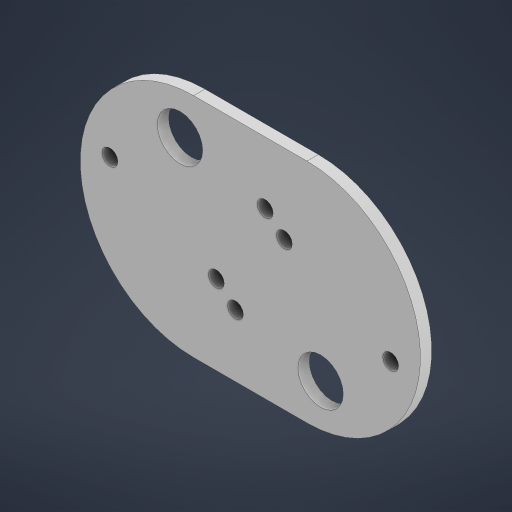
# Autodesk Inventor part: mount-plate
Saved by Autodesk Inventor 2024 (Build 280153000, 153)
## iProperties
Created: 2024-10-23
Part Number: mount-plate
Material: Generic
Document SubType Name: Modeling
Designer: loren
Density: 1 g/cm^3
Appearance: Default
Author: loren
## iProperties of the stored document mount-plate_3DPrint.ipt
Created: 2026-02-06
Part Number: mount-plate_3DPrint
Material: Generic
Document SubType Name: Modeling
Designer: lokies
Density: 1 g/cm^3
Appearance: Default
Author: lokies
Autodesk Inventor part; units mm, degrees
ref_plane "YZ Plane" through (0, 0, 0) normal (1, 0, 0) x (0, 1, 0)
ref_plane "XZ Plane" through (0, 0, 0) normal (0, 1, 0) x (-1, 0, 0)
ref_plane "XY Plane" through (0, 0, 0) normal (0, 0, 1) x (1, 0, 0)
sketch "Sketch1" plane through (0, 0, 0) normal (0, 1, 0) x (-1, 0, 0)
  line L0 (37.5, 25) -> (-37.5, 25)
  line L1 (-37.5, 25) -> (-37.5, -25)
  line L2 (-37.5, -25) -> (37.5, -25)
  line L3 (37.5, -25) -> (37.5, 25)
  circle A0 centre (-7.5, 7.5) radius 1.75
  circle A1 centre (7.5, -7.5) radius 1.75
  line L4 (-7.5, 7.5) -> (7.5, -7.5) construction
  circle A2 centre (15.5, 15.5) radius 5
  line L5 (15.5, 15.5) -> (-15.5, -15.5) construction
  circle A3 centre (-15.5, -15.5) radius 5
  line L6 (15.5, 15.5) -> (13.8367, 7.6748) construction
  line L7 (30.9543, 4.0364) -> (-3.2809, 11.3133) construction
  circle A4 centre (13.8367, 7.6748) radius 14 construction
  line L8 (18.715, -5.4478) -> (4.0428, -2.3291) construction
  line L9 (4.0428, -2.3291) -> (2.9037, -7.6878) construction
  line L10 (2.9037, -7.6878) -> (17.5759, -10.8065) construction
  line L11 (17.5759, -10.8065) -> (18.715, -5.4478) construction
  circle A5 centre (-3.2809, 11.3133) radius 1.75
  circle A6 centre (30.9543, 4.0364) radius 1.75
  line L12 (3.2809, -11.3133) -> (-30.9543, -4.0364) construction
  line L13 (-13.8367, -7.6748) -> (-15.5, -15.5) construction
  circle A7 centre (3.2809, -11.3133) radius 1.75
  circle A8 centre (-30.9543, -4.0364) radius 1.75
  circle A9 centre (-13.8367, -7.6748) radius 14 construction
  line L14 (-4.0428, 2.3291) -> (-18.715, 5.4478) construction
  line L15 (-18.715, 5.4478) -> (-17.5759, 10.8065) construction
  line L16 (-17.5759, 10.8065) -> (-2.9037, 7.6878) construction
  line L17 (-2.9037, 7.6878) -> (-4.0428, 2.3291) construction
  point P0 (0, 0)
  point P1 (0, 0)
  point P2 (0, 25)
  point P3 (-37.5, 0)
  dimension "d0" = 7.5
  dimension "d1" = 7.5
  dimension "d4" = 3.5
  dimension "d6" = 10
  dimension "d7" = 15.5
  dimension "d8" = 15.5
  dimension "d9" = 8
  dimension "d10" = 35
  dimension "d11" = 28
  dimension "d12" = 3.3
  dimension "d13" = 15
  dimension "d14" = 12
  dimension "d15" = 75
  dimension "d16" = 50
  constraints: 36 end point, 13 parallel, 10 centre point, 8 coincident, 7 equal radius, 6 midpoint, 5 perpendicular, 4 point on circle, 1 horizontal, 1 horizontal alignment, 1 vertical alignment
  measures "d0" horizontal distance of point (0, 0) L4.start
  measures "d1" horizontal distance of L4.start point (0, 0)
  measures "d4" diameter of A0
  measures "d6" diameter of A2
  measures "d7" horizontal distance of point (0, 0) L5.start
  measures "d8" horizontal distance of point (0, 0) L5.start
  measures "d9" distance of L5.start L6.end
  measures "d10" distance of L7.start L7.end
  measures "d11" diameter of A4
  measures "d12" distance edge to line of A4 L10
  measures "d13" distance between parallel lines of L9 L11
  measures "d14" angle of L0 L7
  measures "d15" distance of L0.start L0.end
  measures "d16" distance of L0.end L1.end
extrude "Extrusion1" add sketch "Sketch1" along normal blind 2.5
fillet "Fillet1" radius 25 4 edges at (-37.5, 1.25, 25) (37.5, 1.25, 25) (37.5, 1.25, -25) (-37.5, 1.25, -25)
equation "\"d1\" = d0"
equation "\"d8\" = d7"
equation "\"thumbscrew_dia\" = 15.8"
equation "\"helix_length\" = 3.5"
equation "\"helix_width\" = 2"
equation "\"helix_fillet\" = 0.3"
equation "\"helix_inner_dia\" = 19"
equation "\"helix_outer_dia\" = 23"
equation "\"elephant_prevention_radius\" = 0.3"
equation "\"gear_center_distance\" = 25"
equation "\"stepper_screw_dist\" = 35"
equation "\"stepper_axis_offset\" = 8"
equation "\"mount_screw_ortho_dist\" = 31"
equation "\"stepper_dia\" = 28"
equation "\"sheet_thick\" = 2.5"
equation "\"helix_winding_factor\" = 1.2"
body "Solid1"
